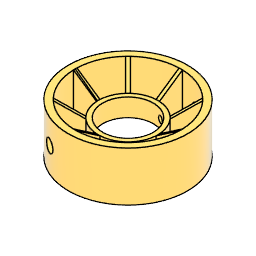
Car5.2 (Autodesk Fusion 360 archive; units mm, degrees)
design "Frontwheel-v1"
Autodesk Fusion 360 part; units mm, degrees
sketch "Sketch1" plane through (0, 0, 0) normal (0, 1, 0) x (1, 0, 0)
  line L0 (-23.488, -0.75) -> (-13.2288, -0.75)
  line L1 (9.8845, -8.8238) -> (17.1389, -16.0782)
  line L2 (0.75, 23.488) -> (0.75, 13.2288)
  line L3 (13.2288, 0.75) -> (23.488, 0.75)
  line L4 (-8.8238, -9.8845) -> (-16.0782, -17.1389)
  line L5 (13.2288, -0.75) -> (23.488, -0.75)
  circle A0 centre (0, 0) radius 26.5
  line L6 (-9.8845, -8.8238) -> (-17.1389, -16.0782)
  line L7 (9.8845, 8.8238) -> (17.1389, 16.0782)
  line L8 (0.75, -13.2288) -> (0.75, -23.488)
  line L9 (-23.488, 0.75) -> (-13.2288, 0.75)
  line L10 (8.8238, 9.8845) -> (16.0782, 17.1389)
  line L11 (8.8238, -9.8845) -> (16.0782, -17.1389)
  line L12 (-9.8845, 8.8238) -> (-17.1389, 16.0782)
  line L13 (-8.8238, 9.8845) -> (-16.0782, 17.1389)
  line L14 (-0.75, 23.488) -> (-0.75, 13.2288)
  line L15 (-0.75, -13.2288) -> (-0.75, -23.488)
  circle A1 centre (0, 0) radius 13.25
  circle A2 centre (0, 0) radius 11.25
  circle A3 centre (0, 0) radius 23.5
  dimension "d2" = 2
  dimension "d4" = 22.5
  constraint coincident A0.centre A1.centre
  constraint coincident L14.start A3
  constraint concentric A0 A3
  constraint coincident L0.start A3
  constraint collinear L3 L9
  constraint collinear L0 L5
  constraint collinear L2 L8
  constraint coincident L12.end A3
  constraint coincident L10.end A3
  constraint coincident L1.end A3
  constraint collinear L14 L15
  constraint coincident A1 L2.end
  constraint coincident A1 L14.end
  constraint coincident A1 L13.start
  constraint coincident A1 L12.start
  constraint coincident A1 L9.end
  constraint coincident A1 L0.end
  constraint coincident A1 L6.start
  constraint coincident A1 L4.start
  constraint coincident A1 L15.start
  constraint coincident A1 L8.start
  constraint coincident A1 L11.start
  constraint coincident A1 L1.start
  constraint coincident A1 L5.start
  constraint coincident A1 L3.start
  constraint coincident A1 L7.start
  constraint coincident A1 L10.start
  constraint coincident L13.end A3
  measures "d4" diameter of A2
extrude "Extrude1" add sketch "Sketch1" along normal mid plane 8 contours A1 makes body 1
extrude "Extrude2" add sketch "Sketch1" along normal mid plane 22 separate body contours L0 L9 A1 A3 | L4 L6 A1 A3 | L12 L13 A1 A3 | L8 L15 A1 A3 | L2 L14 A1 A3 | L1 L11 A1 A3 | L7 L10 A1 A3 | L3 L5 A1 A3 | A0 makes body 2
sketch "Sketch3" plane through (0, 0, 0.75) normal (0, 0, 1) x (1, 0, 0)
  line L0 (-13.2288, -11) -> (-13.2288, 11)
  line L1 (-13.2288, 11) -> (-23.488, 11)
  line L2 (-23.488, 11) -> (-23.488, -11)
  line L3 (-23.488, -11) -> (-13.2288, -11)
  line L4 (13.25, 4) -> (-13.25, 4)
  line L5 (-13.25, 4) -> (-23.488, 11)
  line L6 (-13.25, -4) -> (13.25, -4)
  line L7 (-13.25, -4) -> (-23.488, -11)
  constraint coincident L4.end L5.start
  constraint coincident L1.end L2.start
  constraint coincident L6.start L7.start
  constraint coincident L2.end L3.start
sketch "Sketch13" plane through (0, 11, 0) normal (0, 1, 0) x (-1, 0, 0)
  arc A0 (-13.2288, 0.75) -> (-13.2288, -0.75) centre (0, 0) ccw
  line L0 (-13.2288, 0.75) -> (-23.488, 0.75)
  arc A1 (-17.1389, 16.0782) -> (-23.488, 0.75) centre (0, 0) ccw
  line L1 (-17.1389, 16.0782) -> (-9.8845, 8.8238)
  arc A2 (-8.8238, 9.8845) -> (-9.8845, 8.8238) centre (0, 0) ccw
  line L2 (-8.8238, 9.8845) -> (-16.0782, 17.1389)
  arc A3 (-0.75, 23.488) -> (-16.0782, 17.1389) centre (0, 0) ccw
  line L3 (-0.75, 23.488) -> (-0.75, 13.2288)
  arc A4 (0.75, 13.2288) -> (-0.75, 13.2288) centre (0, 0) ccw
  line L4 (0.75, 13.2288) -> (0.75, 23.488)
  arc A5 (16.0782, 17.1389) -> (0.75, 23.488) centre (0, 0) ccw
  line L5 (16.0782, 17.1389) -> (8.8238, 9.8845)
  arc A6 (9.8845, 8.8238) -> (8.8238, 9.8845) centre (0, 0) ccw
  line L6 (9.8845, 8.8238) -> (17.1389, 16.0782)
  arc A7 (23.488, 0.75) -> (17.1389, 16.0782) centre (0, 0) ccw
  line L7 (23.488, 0.75) -> (13.2288, 0.75)
  arc A8 (13.2288, -0.75) -> (13.2288, 0.75) centre (0, 0) ccw
  line L8 (13.2288, -0.75) -> (23.488, -0.75)
  arc A9 (17.1389, -16.0782) -> (23.488, -0.75) centre (0, 0) ccw
  line L9 (17.1389, -16.0782) -> (9.8845, -8.8238)
  arc A10 (8.8238, -9.8845) -> (9.8845, -8.8238) centre (0, 0) ccw
  line L10 (8.8238, -9.8845) -> (16.0782, -17.1389)
  arc A11 (0.75, -23.488) -> (16.0782, -17.1389) centre (0, 0) ccw
  line L11 (0.75, -23.488) -> (0.75, -13.2288)
  arc A12 (-0.75, -13.2288) -> (0.75, -13.2288) centre (0, 0) ccw
  line L12 (-0.75, -13.2288) -> (-0.75, -23.488)
  arc A13 (-16.0782, -17.1389) -> (-0.75, -23.488) centre (0, 0) ccw
  line L13 (-16.0782, -17.1389) -> (-8.8238, -9.8845)
  arc A14 (-9.8845, -8.8238) -> (-8.8238, -9.8845) centre (0, 0) ccw
  line L14 (-9.8845, -8.8238) -> (-17.1389, -16.0782)
  arc A15 (-23.488, -0.75) -> (-17.1389, -16.0782) centre (0, 0) ccw
  line L15 (-23.488, -0.75) -> (-13.2288, -0.75)
  circle A16 centre (0, 0) radius 26.5
  circle A17 centre (0, 0) radius 23.5
  constraint concentric A0 A17
  constraint coincident A15.start A17
sweep "Sweep1" cut profiles "Sketch3" path "Sketch13" along A17 section 1 contours L0 L3 L6 L7 | L0 L1 L4 L5 bodies 2
combine "Combine1" operation add target body 2 tool bodies 1
ref_plane "WorkPlane1" through (4.7324, 0.5191, -12.3761) normal (0.357159, 0, -0.934044) x (0.934044, 0, 0.357159)
sketch "Sketch14" plane through (4.7324, 0, -12.3761) normal (0.357159, 0, -0.934044) x (0.934044, 0, 0.357159)
  circle A0 centre (0, 0) radius 1.45
  dimension "d16" = 2.9
  constraint coincident A0.centre origin
  measures "d16" diameter of A0
extrude "Extrude3" cut sketch "Sketch14" along normal blind 3 and the other way blind 3 bodies 2
sketch "Sketch15" plane through (4.7324, 0, -12.3761) normal (0.357159, 0, -0.934044) x (0.934044, 0, 0.357159)
  circle A0 centre (0, 0) radius 2.75
  dimension "d21" = 5.5
  constraint coincident A0.centre origin
  measures "d21" diameter of A0
extrude "Extrude4" cut sketch "Sketch15" along normal blind 27 bodies 2
ref_plane "WorkPlane2" through (-5.3818, 0.1633, 12.1078) normal (-0.40617, 0, 0.913797) x (-0.913797, 0, -0.40617)
sketch "Sketch16" plane through (-5.3818, 0, 12.1078) normal (-0.40617, 0, 0.913797) x (-0.913797, 0, -0.40617)
  circle A0 centre (0, 0) radius 1.45
  dimension "d25" = 2.9
  constraint coincident A0.centre origin
  measures "d25" diameter of A0
extrude "Extrude5" cut sketch "Sketch16" against normal blind 4 bodies 2
sketch "Sketch17" plane through (-5.3818, 0, 12.1078) normal (-0.40617, 0, 0.913797) x (-0.913797, 0, -0.40617)
  circle A0 centre (0, 0) radius 2.75
  dimension "d28" = 5.5
  constraint coincident A0.centre origin
  measures "d28" diameter of A0
extrude "Extrude6" cut sketch "Sketch17" along normal blind 22 bodies 2
ref_plane "WorkPlane3" through (26.5, 1.185, 0) normal (1, 0, 0) x (0, 0, 1)

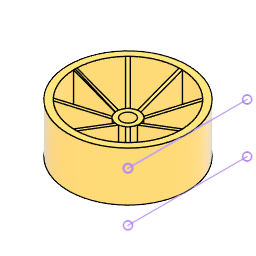
design "Backwheel-v2"
Autodesk Fusion 360 part; units mm, degrees
sketch "Sketch1" plane through (0, 0, 0) normal (0, 1, 0) x (1, 0, 0)
  line L0 (-23.488, -0.75) -> (-4.9434, -0.75)
  line L1 (4.0259, -2.9652) -> (17.1389, -16.0782)
  line L2 (0.75, 23.488) -> (0.75, 4.9434)
  line L3 (4.9434, 0.75) -> (23.488, 0.75)
  line L4 (-2.9652, -4.0259) -> (-16.0782, -17.1389)
  line L5 (4.9434, -0.75) -> (23.488, -0.75)
  circle A0 centre (0, 0) radius 26.5
  line L6 (-4.0259, -2.9652) -> (-17.1389, -16.0782)
  line L7 (4.0259, 2.9652) -> (17.1389, 16.0782)
  line L8 (0.75, -4.9434) -> (0.75, -23.488)
  line L9 (-23.488, 0.75) -> (-4.9434, 0.75)
  line L10 (2.9652, 4.0259) -> (16.0782, 17.1389)
  line L11 (2.9652, -4.0259) -> (16.0782, -17.1389)
  line L12 (-4.0259, 2.9652) -> (-17.1389, 16.0782)
  line L13 (-2.9652, 4.0259) -> (-16.0782, 17.1389)
  line L14 (-0.75, 23.488) -> (-0.75, 4.9434)
  line L15 (-0.75, -4.9434) -> (-0.75, -23.488)
  circle A1 centre (0, 0) radius 5
  circle A2 centre (0, 0) radius 3
  circle A3 centre (0, 0) radius 23.5
  dimension "d2" = 2
  dimension "d4" = 6
  constraint coincident A0.centre A1.centre
  constraint coincident L14.start A3
  constraint concentric A0 A3
  constraint coincident L0.start A3
  constraint collinear L3 L9
  constraint collinear L0 L5
  constraint collinear L2 L8
  constraint coincident L12.end A3
  constraint coincident L10.end A3
  constraint coincident L1.end A3
  constraint collinear L14 L15
  constraint coincident A1 L2.end
  constraint coincident A1 L14.end
  constraint coincident A1 L13.start
  constraint coincident A1 L12.start
  constraint coincident A1 L9.end
  constraint coincident A1 L0.end
  constraint coincident A1 L6.start
  constraint coincident A1 L4.start
  constraint coincident A1 L15.start
  constraint coincident A1 L8.start
  constraint coincident A1 L11.start
  constraint coincident A1 L1.start
  constraint coincident A1 L5.start
  constraint coincident A1 L3.start
  constraint coincident A1 L7.start
  constraint coincident A1 L10.start
  constraint coincident L13.end A3
  measures "d4" diameter of A2
extrude "Extrude1" add sketch "Sketch1" along normal mid plane 8 contours A1 makes body 1
extrude "Extrude2" add sketch "Sketch1" along normal mid plane 22 separate body contours L0 L9 A1 A3 | L4 L6 A1 A3 | L12 L13 A1 A3 | L8 L15 A1 A3 | L2 L14 A1 A3 | L1 L11 A1 A3 | L7 L10 A1 A3 | L3 L5 A1 A3 | A0 makes body 2
sketch "Sketch3" plane through (0, 0, 0.75) normal (0, 0, 1) x (1, 0, 0)
  line L0 (-4.9434, -11) -> (-4.9434, 11)
  line L1 (-4.9434, 11) -> (-23.488, 11)
  line L2 (-23.488, 11) -> (-23.488, -11)
  line L3 (-23.488, -11) -> (-4.9434, -11)
  line L4 (5, 4) -> (-5, 4)
  line L5 (-5, 4) -> (-23.488, 11)
  line L6 (-5, -4) -> (5, -4)
  line L7 (-5, -4) -> (-23.488, -11)
  constraint coincident L4.end L5.start
  constraint coincident L1.end L2.start
  constraint coincident L6.start L7.start
  constraint coincident L2.end L3.start
sketch "Sketch13" plane through (0, 11, 0) normal (0, 1, 0) x (-1, 0, 0)
  arc A0 (-4.9434, 0.75) -> (-4.9434, -0.75) centre (0, 0) ccw
  line L0 (-4.9434, 0.75) -> (-23.488, 0.75)
  arc A1 (-17.1389, 16.0782) -> (-23.488, 0.75) centre (0, 0) ccw
  line L1 (-17.1389, 16.0782) -> (-4.0259, 2.9652)
  arc A2 (-2.9652, 4.0259) -> (-4.0259, 2.9652) centre (0, 0) ccw
  line L2 (-2.9652, 4.0259) -> (-16.0782, 17.1389)
  arc A3 (-0.75, 23.488) -> (-16.0782, 17.1389) centre (0, 0) ccw
  line L3 (-0.75, 23.488) -> (-0.75, 4.9434)
  arc A4 (0.75, 4.9434) -> (-0.75, 4.9434) centre (0, 0) ccw
  line L4 (0.75, 4.9434) -> (0.75, 23.488)
  arc A5 (16.0782, 17.1389) -> (0.75, 23.488) centre (0, 0) ccw
  line L5 (16.0782, 17.1389) -> (2.9652, 4.0259)
  arc A6 (4.0259, 2.9652) -> (2.9652, 4.0259) centre (0, 0) ccw
  line L6 (4.0259, 2.9652) -> (17.1389, 16.0782)
  arc A7 (23.488, 0.75) -> (17.1389, 16.0782) centre (0, 0) ccw
  line L7 (23.488, 0.75) -> (4.9434, 0.75)
  arc A8 (4.9434, -0.75) -> (4.9434, 0.75) centre (0, 0) ccw
  line L8 (4.9434, -0.75) -> (23.488, -0.75)
  arc A9 (17.1389, -16.0782) -> (23.488, -0.75) centre (0, 0) ccw
  line L9 (17.1389, -16.0782) -> (4.0259, -2.9652)
  arc A10 (2.9652, -4.0259) -> (4.0259, -2.9652) centre (0, 0) ccw
  line L10 (2.9652, -4.0259) -> (16.0782, -17.1389)
  arc A11 (0.75, -23.488) -> (16.0782, -17.1389) centre (0, 0) ccw
  line L11 (0.75, -23.488) -> (0.75, -4.9434)
  arc A12 (-0.75, -4.9434) -> (0.75, -4.9434) centre (0, 0) ccw
  line L12 (-0.75, -4.9434) -> (-0.75, -23.488)
  arc A13 (-16.0782, -17.1389) -> (-0.75, -23.488) centre (0, 0) ccw
  line L13 (-16.0782, -17.1389) -> (-2.9652, -4.0259)
  arc A14 (-4.0259, -2.9652) -> (-2.9652, -4.0259) centre (0, 0) ccw
  line L14 (-4.0259, -2.9652) -> (-17.1389, -16.0782)
  arc A15 (-23.488, -0.75) -> (-17.1389, -16.0782) centre (0, 0) ccw
  line L15 (-23.488, -0.75) -> (-4.9434, -0.75)
  circle A16 centre (0, 0) radius 26.5
  circle A17 centre (0, 0) radius 23.5
  constraint concentric A0 A17
  constraint coincident A15.start A17
sweep "Sweep1" cut profiles "Sketch3" path "Sketch13" along A17 section 1 contours L0 L3 L6 L7 | L0 L1 L4 L5 bodies 2
combine "Combine1" operation add target body 2 tool bodies 1
move_body "Move1" bodies 2 to x (1, 0, 0) y (0, 1, 0) z (0, 0, 1) at (0.4999, 0, 0.0077)
ref_plane "WorkPlane1" through (26.9999, 2.9703, 0.0077) normal (1, 0, 0) x (0, 0, 1)
sketch "Sketch14" plane through (26.9999, 0, 0) normal (1, 0, 0) x (0, 0, -1)
  line L0 (-26.5077, -11) -> (26.4923, -11)
  line L1 (26.4923, 11) -> (-26.5077, 11)
